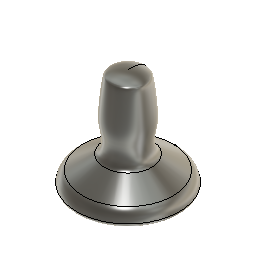
Joystick_originale (Autodesk Fusion 360 design; units mm, degrees)
Autodesk Fusion 360 part; units mm, degrees
sketch "Schizzo1" plane through (0, 0, 0) normal (1, 0, 0) x (0, 1, 0)
  line L0 (3.225, 0) -> (3.225, 15)
  line L1 (3.225, 15) -> (0, 15)
  line L2 (0, 0) -> (0, 15) construction
  line L3 (0, 0) -> (3.225, 0) construction
  line L4 (3.225, 0) -> (6.5, 0)
  circle A0 centre (20.25, -9.5) radius 1.5
  line L5 (20.25, -11) -> (20.25, -9.5) construction
  line L6 (20.25, -9.5) -> (21.75, -9.5) construction
  line L7 (6.5, 0) -> (7.3213, -3.4454)
  line L8 (7.3213, -3.4454) -> (13.5404, -2.9191)
  line L9 (13.5404, -2.9191) -> (18, -7)
  line L10 (18, -7) -> (18.8346, -9.0034)
  spline S0 degree 4 poles (6.5, 0) (7.3213, -3.4454) (13.5404, -2.9191) (18, -7) (18.8346, -9.0034) knots 0 0 0 0 0 1 1 1 1 1
  line L11 (10, 1) -> (19.0622, -4.9101)
  line L12 (21.7446, -9.3727) -> (21.5, -6.5)
  line L13 (21.5, -6.5) -> (19.0622, -4.9101)
  spline S1 degree 2 poles (21.7446, -9.3727) (21.5, -6.5) (19.0622, -4.9101) knots 0 0 0 1 1 1
  line L14 (0, 15) -> (0, 32)
  line L15 (0, 30) -> (7.25, 30) construction
  line L16 (0, 15) -> (9, 15) construction
  line L17 (0, 6) -> (8, 6) construction
  spline S2 degree 5 poles (0, 32) (0.6347, 32) (1.823, 31.9581) (3.3621, 31.77) (4.944, 31.3305) (6.2411, 30.754) (7.0133, 30.3055) (7.4444, 29.9081) (7.7573, 28.7514) (8.0621, 26.6267) (8.3862, 23.7438) (8.701, 20.5398) (8.9436, 17.4811) (9.0489, 14.9377) (8.9557, 12.8641) (8.6827, 10.9978) (8.3415, 9.2705) (8.0576, 7.6242) (7.9527, 6.0601) (8.0382, 4.5556) (8.3134, 3.129) (8.7776, 2.1325) (9.3099, 1.511) (9.755, 1.1598) (10, 1) knots 0 0 0 0 0 0 0.05 0.1 0.15 0.2 0.25 0.3 0.35 0.4 0.45 0.5 0.55 0.6 0.65 0.7 0.75 0.8 0.85 0.9 0.95 1 1 1 1 1 1
  line L18 (-7, 32) -> (7, 32)
  line L19 (6.5, 31) -> (8, 29)
  line L20 (9, 19) -> (9, 11)
  line L21 (8, 9.4368) -> (8, 2.5632)
  point P0 (20.25, -11)
  dimension "d1" = 3.225
  dimension "d2" = 15
  dimension "d3" = 6.5
  dimension "d5" = 11
  dimension "d6" = 3
  dimension "d7" = 21.75
  dimension "d8" = 10
  dimension "d9" = 1
  dimension "d10" = 31
  dimension "d11" = 7.25
  dimension "d12" = 2
  dimension "d13" = 9
  dimension "d14" = 14
  dimension "d15" = 8
  dimension "d16" = 5
  constraint vertical L0
  constraint perpendicular L0 L1
  constraint coincident L2.start L3.start
  constraint perpendicular L1 L2
  constraint perpendicular L0 L3
  constraint perpendicular L0 L4
  constraint coincident P0 A0
  constraint coincident P0 L5.start
  constraint coincident A0.centre L5.end
  constraint vertical L5
  constraint coincident A0 L6.end
  constraint perpendicular L5 L6
  constraint coincident A0 L10.end
  constraint coincident A0 L12.start
  constraint tangent A0 S1
  constraint perpendicular L1 L14
  constraint coincident L14 L15.start
  constraint perpendicular L14 L15
  constraint coincident L14 L1.end
  constraint perpendicular L14 L16
  constraint coincident L2 L17.start
  constraint perpendicular L2 L17
  constraint midpoint L14.end L18
  constraint horizontal L18
  constraint midpoint L15.end L19
  constraint midpoint L16.end L20
  constraint vertical L20
  constraint midpoint L17.end L21
  constraint vertical L21
  measures "d1" distance of L0 L2
  measures "d2" distance of L0.start L0.end
  measures "d3" distance of L2.start L4.end
  measures "d5" distance of L4 P0
  measures "d6" diameter of A0
  measures "d7" distance of L2 L6.end
  measures "d8" distance of L2 L11.start
  measures "d9" vertical distance of L4.end L11.start
  measures "d10" vertical distance of L11.start L14.end
  measures "d11" distance of L15.start L15.end
  measures "d12" distance of L14.end L15
  measures "d13" distance of L1.end L16.end
  measures "d14" vertical distance of L11.start L16.end
  measures "d15" distance of L17.start L17.end
  measures "d16" distance of L11.start L17
revolve "Rivoluzione1" add sketch "Schizzo1" angle 360 about axis through (0, 0, 0) along (0, 0, 1) contours L0 L1 L4 A0 L8 L9 L10 S0 L11 S1 L14 S2 | L8 L9 L10 S0 | A0
chamfer "Smusso1" distance 1 angle 45 1 edges at (-3.0068, 1.1662, 0)
equation "d1 = ( larghezza_incastro_joystick / 2 )"
equation "d3 = ( 13 / 2 ) * 1 mm"
equation "d7 = ( 43.5 / 2 ) * 1 mm"
equation "d8 = ( 20 / 2 ) * 1 mm"
equation "d11 = ( 14.5 / 2 ) * 1 mm"
equation "d13 = ( 18 / 2 ) * 1 mm"
equation "d15 = ( 16 / 2 ) * 1 mm"
equation "larghezza_incastro_joystick = 6.45 mm" comment "Modificare questo valore per allargare o diminuire il foro dell'incastro del Joystick. (Valore di default 6.45 mm)"
named bodies: "joystick"
